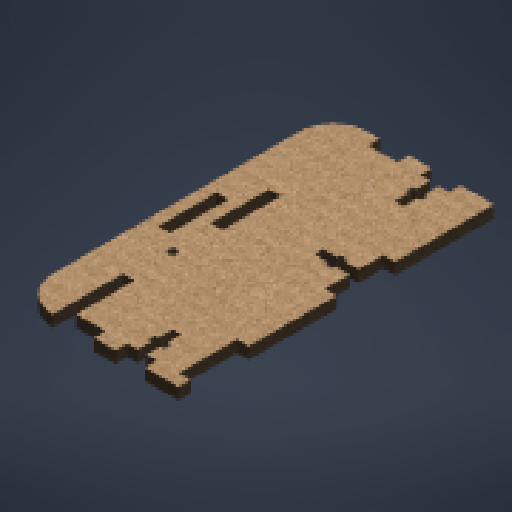
# Autodesk Inventor part: FloorButtonHolder_Bottom_V1_B
Saved by Autodesk Inventor 2024.1 (Build 281209000, 209)
## iProperties
Created: 2023-05-20
Part Number: FloorButtonHolder_Bottom_V1_B
Material: MDF Medium Density Fiberboard
Document SubType Name: Modeling
Designer: jaege
Density: 0.8 g/cm^3
Appearance: Cardboard - Corrugated
Author: jaege
Autodesk Inventor part; units mm, degrees
ref_plane "YZ Plane" through (0, 0, 0) normal (1, 0, 0) x (0, 1, 0)
ref_plane "XZ Plane" through (0, 0, 0) normal (0, 1, 0) x (-1, 0, 0)
ref_plane "XY Plane" through (0, 0, 0) normal (0, 0, 1) x (1, 0, 0)
sketch "Sketch1" plane through (0, 0, 0) normal (0, 1, 0) x (-1, 0, 0)
  line L0 (-17.5, 50) -> (17.5, 50)
  line L1 (17.5, 50) -> (17.5, -50)
  line L2 (17.5, -50) -> (-17.5, -50)
  line L3 (-17.5, -50) -> (-17.5, 50)
  line L4 (-17.5, 50) -> (17.5, -50) construction
  line L5 (17.5, 50) -> (-17.5, -50) construction
  line L6 (7.5, 50) -> (0, 50)
  line L7 (0, 50) -> (0, 54)
  line L8 (0, 54) -> (7.5, 54)
  line L9 (7.5, 54) -> (7.5, 50)
  line L10 (-10, 50) -> (-21.5, 50)
  line L11 (-21.5, 50) -> (-21.5, 54)
  line L12 (-21.5, 54) -> (-10, 54)
  line L13 (-10, 54) -> (-10, 50)
  line L14 (17.5, 30) -> (21.5, 30)
  line L15 (21.5, 30) -> (21.5, 0)
  line L16 (21.5, 0) -> (17.5, 0)
  line L17 (17.5, 0) -> (17.5, 30)
  line L18 (17.5, -20) -> (21.5, -20)
  line L19 (21.5, -20) -> (21.5, -54)
  line L20 (21.5, -54) -> (17.5, -54)
  line L21 (17.5, -54) -> (17.5, -20)
  line L22 (7.5, -50) -> (0, -50)
  line L23 (0, -50) -> (0, -54)
  line L24 (0, -54) -> (7.5, -54)
  line L25 (7.5, -54) -> (7.5, -50)
  line L26 (-10, -50) -> (-21.5, -50)
  line L27 (-21.5, -50) -> (-21.5, -54)
  line L28 (-21.5, -54) -> (-10, -54)
  line L29 (-10, -54) -> (-10, -50)
  line L30 (-17.5, 30) -> (-21.5, 30)
  line L31 (-21.5, 30) -> (-21.5, 0)
  line L32 (-21.5, 0) -> (-17.5, 0)
  line L33 (-17.5, 0) -> (-17.5, 30)
  line L34 (-17.5, -50) -> (-21.5, -50)
  line L35 (-21.5, -50) -> (-21.5, -20)
  line L36 (-21.5, -20) -> (-17.5, -20)
  line L37 (-17.5, -20) -> (-17.5, -50)
  point P0 (0, 0)
  point P1 (17.5, 0)
  point P2 (-17.5, 50)
  point P3 (-17.5, 0)
  point P4 (-21.5, -50)
  point P5 (17.5, -50)
  point P6 (19.5, -54)
  dimension "d0" = 35
  dimension "d2" = 7.5
  dimension "d3" = 4
  dimension "d4" = 11.5
  dimension "d5" = 4
  dimension "d6" = 10
  dimension "d7" = 10
  dimension "d8" = 4
  dimension "d9" = 30
  dimension "d10" = 4
  dimension "d11" = 34
  dimension "d12" = 20
  dimension "d13" = 20
  dimension "d14" = 7.5
  dimension "d15" = 4
  dimension "d16" = 11.5
  dimension "d17" = 4
  dimension "d18" = 10
  dimension "d19" = 10
  dimension "d20" = 4
  dimension "d21" = 30
  dimension "d22" = 20
  dimension "d23" = 4
  dimension "d24" = 30
  dimension "d27" = 4
  constraints: 76 end point, 18 parallel, 9 horizontal, 9 perpendicular, 7 point on line, 3 midpoint
  measures "d0" distance of L1.end L2.end
  measures "d2" distance of L7.end L8.end
  measures "d3" distance of L6.end L7.end
  measures "d4" distance of L11.end L12.end
  measures "d5" distance of L10.end L11.end
  measures "d6" distance between parallel lines of L9 L1
  measures "d7" distance between parallel lines of L13 L7
  measures "d8" distance of L15.end L16.end
  measures "d9" distance of L14.end L15.end
  measures "d10" distance of L19.end L20.end
  measures "d11" distance of L18.end L19.end
  measures "d12" distance between parallel lines of L16 L18
  measures "d13" distance between parallel lines of L0 L14
  measures "d14" distance of L24.end L23.end
  measures "d15" distance of L23.end L22.end
  measures "d16" distance of L28.end L27.end
  measures "d17" distance of L27.end L26.end
  measures "d18" distance between parallel lines of L25 L21
  measures "d19" distance between parallel lines of L29 L23
  measures "d20" distance of L32.end L31.end
  measures "d21" distance of L31.end L30.end
  measures "d22" distance between parallel lines of L10 L30
  measures "d23" distance of L35.end L36.end
  measures "d24" distance of L34.end L35.end
  measures "d27" distance from line of L2 point (19.5, -54)
extrude "Extrusion1" add sketch "Sketch1" along normal blind 4
sketch "Sketch2" plane through (0, 4, 0) normal (0, 1, 0) x (1, 0, 0)
  line L0 (-21.5, 54) -> (-33.5, 54)
  line L1 (-33.5, 54) -> (-33.5, -54)
  line L2 (-33.5, -54) -> (-21.5, -54)
  line L3 (-21.5, -54) -> (-21.5, 54)
  line L4 (-21.5, 54) -> (-21.5, 20) projected
  line L5 (-21.5, 20) -> (-17.5, 20) projected
  line L6 (-17.5, 20) -> (-17.5, 0) projected
  line L7 (-17.5, 0) -> (-21.5, 0) projected
  line L8 (-21.5, 0) -> (-21.5, -30) projected
  line L9 (-21.5, -30) -> (-17.5, -30) projected
  line L10 (-17.5, -30) -> (-17.5, -50) projected
  line L11 (-17.5, -50) -> (-7.5, -50) projected
  line L12 (-7.5, -50) -> (-7.5, -54) projected
  line L13 (-7.5, -54) -> (0, -54) projected
  line L14 (0, -54) -> (0, -50) projected
  line L15 (0, -50) -> (10, -50) projected
  line L16 (10, -50) -> (10, -54) projected
  line L17 (10, -54) -> (21.5, -54) projected
  line L18 (21.5, -54) -> (21.5, -50) projected
  line L19 (21.5, -50) -> (17.5, -50) projected
  line L20 (17.5, -50) -> (17.5, -30) projected
  line L21 (17.5, -30) -> (21.5, -30) projected
  line L22 (21.5, -30) -> (21.5, 0) projected
  line L23 (21.5, 0) -> (17.5, 0) projected
  line L24 (17.5, 0) -> (17.5, 20) projected
  line L25 (17.5, 20) -> (21.5, 20) projected
  line L26 (21.5, 20) -> (21.5, 54) projected
  line L27 (21.5, 54) -> (10, 54) projected
  line L28 (10, 54) -> (10, 50) projected
  line L29 (10, 50) -> (0, 50) projected
  line L30 (0, 50) -> (0, 54) projected
  line L31 (0, 54) -> (-7.5, 54) projected
  line L32 (-7.5, 54) -> (-7.5, 50) projected
  line L33 (-7.5, 50) -> (-17.5, 50) projected
  line L34 (-17.5, 50) -> (-17.5, 54) projected
  line L35 (-17.5, 54) -> (-21.5, 54) projected
  line L36 (-7.5, -54) -> (0, -54) projected
  line L37 (-33.5, 54) -> (21.5, -54) construction
  line L38 (-29.5, 10) -> (-25.5, 10)
  line L39 (-25.5, 10) -> (-25.5, -10)
  line L40 (-25.5, -10) -> (-29.5, -10)
  line L41 (-29.5, -10) -> (-29.5, 10)
  point P0 (0, 0)
  point P1 (-6, 0)
  point P2 (-25.5, 0)
  dimension "d28" = 51
  dimension "d34" = 20
  dimension "d35" = 4
  dimension "d36" = 4
  constraints: 18 end point, 4 parallel, 2 horizontal, 2 midpoint, 2 perpendicular, 1 coincident, 1 collinear, 1 horizontal alignment
  measures "d28" distance between parallel lines of L1 L24
  measures "d34" distance of L38.end L39.end
  measures "d35" distance of L38.start L38.end
  measures "d36" distance between parallel lines of L1 L41
extrude "Extrusion2" add sketch "Sketch2" against normal up to surface (4 mm away) contours L3 L2 L1 L0
sketch "Sketch3" plane through (0, 4, 0) normal (0, 1, 0) x (1, 0, 0)
  line L0 (3.5, 45.2) -> (3.5, 50) projected
  line L1 (3.5, 50) -> (0, 50) projected
  line L2 (0, 50) -> (0, 54) construction
  line L3 (0, 54) -> (-7.5, 54) construction
  line L4 (-7.5, 54) -> (-7.5, 50) construction
  line L5 (-7.5, 50) -> (-17.5, 50) construction
  line L6 (-17.5, 50) -> (-17.5, 54) construction
  line L7 (-17.5, 54) -> (-21.5, 54) construction
  line L8 (-17.5, 0) -> (-21.5, 0) construction
  line L9 (-21.5, 0) -> (-21.5, -30) construction
  line L10 (-21.5, -30) -> (-17.5, -30) construction
  line L11 (-17.5, -30) -> (-17.5, -50) construction
  line L12 (-17.5, -50) -> (-7.5, -50) construction
  line L13 (-7.5, -50) -> (-7.5, -54) construction
  line L14 (-7.5, -54) -> (0, -54) construction
  line L15 (0, -54) -> (0, -50) construction
  line L16 (0, -50) -> (3.5, -50) projected
  line L17 (3.5, -50) -> (3.5, -45.2) projected
  line L18 (3.5, -45.2) -> (2.3, -45.2) projected
  line L19 (2.3, -45.2) -> (2.3, -42.8) projected
  line L20 (2.3, -42.8) -> (3.5, -42.8) projected
  line L21 (3.5, -42.8) -> (3.5, -38) projected
  line L22 (3.5, -38) -> (6.5, -38) projected
  line L23 (6.5, -38) -> (6.5, -42.8) projected
  line L24 (6.5, -42.8) -> (7.7, -42.8) projected
  line L25 (7.7, -42.8) -> (7.7, -45.2) projected
  line L26 (7.7, -45.2) -> (6.5, -45.2) projected
  line L27 (6.5, -45.2) -> (6.5, -50) projected
  line L28 (6.5, -50) -> (10, -50) construction
  line L29 (10, -50) -> (10, -54) construction
  line L30 (10, -54) -> (21.5, -54) construction
  line L31 (21.5, -54) -> (21.5, -50) construction
  line L32 (21.5, -50) -> (17.5, -50) construction
  line L33 (17.5, -50) -> (17.5, -30) construction
  line L34 (17.5, -30) -> (21.5, -30) construction
  line L35 (21.5, 0) -> (17.5, 0) construction
  line L36 (17.5, 0) -> (17.5, 8.5) construction
  line L37 (17.5, 8.5) -> (12.7, 8.5) projected
  line L38 (12.7, 8.5) -> (12.7, 7.3) projected
  line L39 (12.7, 7.3) -> (10.3, 7.3) projected
  line L40 (10.3, 7.3) -> (10.3, 8.5) projected
  line L41 (10.3, 8.5) -> (5.5, 8.5) projected
  line L42 (5.5, 8.5) -> (5.5, 11.5) projected
  line L43 (5.5, 11.5) -> (10.3, 11.5) projected
  line L44 (10.3, 11.5) -> (10.3, 12.7) projected
  line L45 (10.3, 12.7) -> (12.7, 12.7) projected
  line L46 (12.7, 12.7) -> (12.7, 11.5) projected
  line L47 (12.7, 11.5) -> (17.5, 11.5) projected
  line L48 (17.5, 11.5) -> (17.5, 20) construction
  line L49 (17.5, 20) -> (21.5, 20) construction
  line L50 (21.5, 20) -> (21.5, 54) construction
  line L51 (21.5, 54) -> (10, 54) construction
  line L52 (10, 54) -> (10, 50) construction
  line L53 (10, 50) -> (6.5, 50) projected
  line L54 (6.5, 50) -> (6.5, 45.2) projected
  line L55 (6.5, 45.2) -> (7.7, 45.2) projected
  line L56 (7.7, 45.2) -> (7.7, 42.8) projected
  line L57 (7.7, 42.8) -> (6.5, 42.8) projected
  line L58 (6.5, 42.8) -> (6.5, 38) projected
  line L59 (6.5, 38) -> (3.5, 38) projected
  line L60 (3.5, 38) -> (3.5, 42.8) projected
  line L61 (3.5, 42.8) -> (2.3, 42.8) projected
  line L62 (2.3, 42.8) -> (2.3, 45.2) projected
  line L63 (2.3, 45.2) -> (3.5, 45.2) projected
  circle A0 centre (-19.5, -15) radius 1.5 projected
  line L64 (-21.5, -30) -> (-17.5, -30) construction
  line L65 (-17.5, -30) -> (-17.5, -50) construction
  line L66 (-17.5, -50) -> (-7.5, -50) construction
  line L67 (-7.5, -50) -> (-7.5, -54) construction
  line L68 (-7.5, -54) -> (0, -54) construction
  line L69 (0, -54) -> (0, -50) construction
  line L70 (0, -50) -> (10, -50) projected
  line L71 (10, -50) -> (10, -54) construction
  line L72 (10, -54) -> (21.5, -54) construction
  line L73 (21.5, -54) -> (21.5, -50) construction
  line L74 (21.5, -50) -> (17.5, -50) construction
  line L75 (17.5, -50) -> (17.5, -30) construction
  line L76 (17.5, -30) -> (21.5, -30) construction
  line L77 (21.5, -30) -> (21.5, 0) construction
  line L78 (21.5, 0) -> (17.5, 0) construction
  line L79 (17.5, 0) -> (17.5, 20) projected
  line L80 (17.5, 20) -> (21.5, 20) construction
  line L81 (21.5, 20) -> (21.5, 54) construction
  line L82 (21.5, 54) -> (10, 54) construction
  line L83 (10, 54) -> (10, 50) construction
  line L84 (10, 50) -> (0, 50) projected
  line L85 (0, 50) -> (0, 54) construction
  line L86 (0, 54) -> (-7.5, 54) construction
  line L87 (-7.5, 54) -> (-7.5, 50) construction
  line L88 (-7.5, 50) -> (-17.5, 50) construction
  line L89 (-17.5, 50) -> (-17.5, 54) construction
  line L90 (-17.5, 54) -> (-33.5, 54) construction
  line L91 (-33.5, 54) -> (-33.5, -54) construction
  line L92 (-33.5, -54) -> (-21.5, -54) construction
  line L93 (-21.5, -54) -> (-21.5, -30) construction
  line L94 (-29.5, 10) -> (-25.5, 10) construction
  line L95 (-25.5, 10) -> (-25.5, -10) construction
  line L96 (-25.5, -10) -> (-29.5, -10) construction
  line L97 (-29.5, -10) -> (-29.5, 10) construction
  line L98 (-21.5, 0) -> (-21.5, 20) construction
  line L99 (-21.5, 20) -> (-17.5, 20) construction
  line L100 (-17.5, 20) -> (-17.5, 0) projected
  line L101 (-17.5, 0) -> (-21.5, 0) construction
  point P0 (0, 0)
  point P1 (-17.5, 11.5)
  point P2 (-12.7, 8.5)
extrude "Extrusion3" cut sketch "Sketch3" against normal up to next
fillet "Fillet1" radius 12 2 edges at (-33.5, 2, 54) (-33.5, 2, -54)
body "Solid1"
